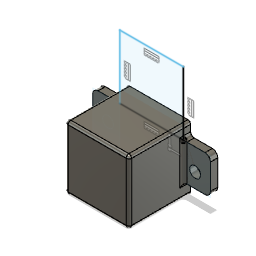
12v ouput cover v1 (Autodesk Fusion 360 design; units mm, degrees)
Autodesk Fusion 360 part; units mm, degrees
sketch "Sketch5" plane through (0, 0, 0) normal (0, 0, 1) x (1, 0, 0)
  line L0 (25.1413, 25.1399) -> (-9.8587, 25.1399)
  line L1 (-9.8587, 25.1399) -> (-9.8587, -9.8601)
  line L2 (-9.8587, -9.8601) -> (25.1413, -9.8601)
  line L3 (25.1413, -9.8601) -> (25.1413, 25.1399)
  line L4 (-9.8587, 18.1399) -> (-24.8587, 18.1399)
  line L5 (-24.8587, 18.1399) -> (-24.8587, -1.8601)
  line L6 (-24.8587, -1.8601) -> (-9.8587, -1.8601)
  line L7 (-9.8587, -1.8601) -> (-9.8587, 18.1399)
  line L8 (25.1413, 18.1399) -> (40.1413, 18.1399)
  line L9 (40.1413, 18.1399) -> (40.1413, -1.8601)
  line L10 (40.1413, -1.8601) -> (25.1413, -1.8601)
  line L11 (25.1413, -1.8601) -> (25.1413, 18.1399)
  dimension "d12" = 35
  dimension "d13" = 35
  dimension "d14" = 15
  dimension "d15" = 20
  dimension "d16" = 7
  dimension "d17" = 15
  dimension "d18" = 20
  dimension "d19" = 7
  constraint horizontal L0
  constraint vertical L1
  constraint horizontal L2
  constraint vertical L3
  constraint horizontal L4
  constraint vertical L5
  constraint horizontal L6
  constraint vertical L7
  constraint coincident L1 L4.start
  constraint horizontal L8
  constraint vertical L9
  constraint horizontal L10
  constraint vertical L11
  constraint coincident L3 L8.start
  measures "d12" distance of L0.start L0.end
  measures "d13" distance of L0.start L2.end
  measures "d14" distance of L4.start L4.end
  measures "d15" distance of L4.start L6.end
  measures "d16" distance of L0 L4
  measures "d17" distance of L8.start L8.end
  measures "d18" distance of L8.start L10.end
  measures "d19" distance of L0 L8
extrude "Extrude4" add sketch "Sketch5" along normal blind 4
sketch "Sketch6" plane through (0, 0, 4) normal (0, 0, 1) x (1, 0, 0)
  line L0 (25.1413, 18.1399) -> (25.1413, 25.1399)
  line L1 (25.1413, 25.1399) -> (-9.8587, 25.1399)
  line L2 (-9.8587, 25.1399) -> (-9.8587, 18.1399)
  line L3 (-9.8587, 18.1399) -> (-24.8587, 18.1399)
  line L4 (-24.8587, 18.1399) -> (-24.8587, -1.8601)
  line L5 (-24.8587, -1.8601) -> (-9.8587, -1.8601)
  line L6 (-9.8587, -1.8601) -> (-9.8587, -9.8601)
  line L7 (-9.8587, -9.8601) -> (25.1413, -9.8601)
  line L8 (25.1413, -9.8601) -> (25.1413, -1.8601)
  line L9 (25.1413, -1.8601) -> (40.1413, -1.8601)
  line L10 (40.1413, -1.8601) -> (40.1413, 18.1399)
  line L11 (40.1413, 18.1399) -> (25.1413, 18.1399)
  circle A0 centre (-16.3587, 6.1399) radius 3
  circle A1 centre (31.6413, 6.1399) radius 3
  line L12 (7.6413, 25.1399) -> (7.6413, -9.8601) construction
  dimension "d22" = 6
  dimension "d23" = 6
  dimension "d24" = 48
  dimension "d25" = 12
  dimension "d26" = 12
  dimension "d27" = 24
  constraint midpoint L1 L12.start
  constraint midpoint L7 L12.end
  measures "d22" diameter of A0
  measures "d23" diameter of A1
  measures "d24" horizontal distance of A0.centre A1.centre
  measures "d25" distance of L3 A0.centre
  measures "d26" distance of L11 A1.centre
  measures "d27" distance of A0.centre L12
extrude "Extrude5" cut sketch "Sketch6" against normal up to surface (4 mm away) contours A0 | A1
sketch "Sketch7" plane through (0, 0, 4) normal (0, 0, 1) x (1, 0, 0)
  circle A0 centre (-16.3587, 6.1399) radius 3
  circle A1 centre (31.6413, 6.1399) radius 3
  line L0 (25.1413, 18.1399) -> (25.1413, 25.1399)
  line L1 (25.1413, 25.1399) -> (-9.8587, 25.1399)
  line L2 (-9.8587, 25.1399) -> (-9.8587, 18.1399)
  line L3 (-9.8587, 18.1399) -> (-24.8587, 18.1399)
  line L4 (-24.8587, 18.1399) -> (-24.8587, -1.8601)
  line L5 (-24.8587, -1.8601) -> (-9.8587, -1.8601)
  line L6 (-9.8587, -1.8601) -> (-9.8587, -9.8601)
  line L7 (-9.8587, -9.8601) -> (25.1413, -9.8601)
  line L8 (25.1413, -9.8601) -> (25.1413, -1.8601)
  line L9 (25.1413, -1.8601) -> (40.1413, -1.8601)
  line L10 (40.1413, -1.8601) -> (40.1413, 18.1399)
  line L11 (40.1413, 18.1399) -> (25.1413, 18.1399)
  line L12 (-5.8587, 21.1399) -> (21.1413, 21.1399)
  line L13 (21.1413, 21.1399) -> (21.1413, -9.8601)
  line L14 (21.1413, -9.8601) -> (-5.8587, -9.8601)
  line L15 (-5.8587, -9.8601) -> (-5.8587, 21.1399)
  dimension "d30" = 4
  dimension "d31" = 4
  dimension "d32" = 4
  constraint coincident L7 L13.end
  measures "d30" distance of L1 L12
  measures "d31" distance of L2 L15
  measures "d32" distance of L0 L13
sketch "Sketch9" plane through (0, 0, 4) normal (0, 0, 1) x (1, 0, 0)
  circle A0 centre (-16.3587, 6.1399) radius 3
  circle A1 centre (31.6413, 6.1399) radius 3
  line L0 (25.1413, 18.1399) -> (25.1413, 25.1399)
  line L1 (25.1413, 25.1399) -> (-9.8587, 25.1399)
  line L2 (-9.8587, 25.1399) -> (-9.8587, 18.1399)
  line L3 (-9.8587, 18.1399) -> (-24.8587, 18.1399)
  line L4 (-24.8587, 18.1399) -> (-24.8587, -1.8601)
  line L5 (-24.8587, -1.8601) -> (-9.8587, -1.8601)
  line L6 (-9.8587, -1.8601) -> (-9.8587, -9.8601)
  line L7 (-9.8587, -9.8601) -> (25.1413, -9.8601)
  line L8 (25.1413, -9.8601) -> (25.1413, -1.8601)
  line L9 (25.1413, -1.8601) -> (40.1413, -1.8601)
  line L10 (40.1413, -1.8601) -> (40.1413, 18.1399)
  line L11 (40.1413, 18.1399) -> (25.1413, 18.1399)
  line L12 (-9.8587, 25.1399) -> (25.1413, 25.1399)
  line L13 (25.1413, 25.1399) -> (25.1413, -9.8601)
  line L14 (25.1413, -9.8601) -> (-9.8587, -9.8601)
  line L15 (-9.8587, -9.8601) -> (-9.8587, 25.1399)
  constraint horizontal L12
  constraint vertical L13
  constraint horizontal L14
  constraint vertical L15
  constraint coincident L7.end L8.start
  constraint coincident L1.end L2.start
extrude "Extrude7" add sketch "Sketch9" along normal blind 30 contours L0 L1 L2 L6 L7 L8 L12 L13 L14 L15
extrude "Extrude6" cut sketch "Sketch7" against normal blind 4 contours L7 L12 L13 L14 L15
sketch "Sketch8" plane through (0, 0, 4) normal (0, 0, 1) x (1, 0, 0)
  line L0 (25.1413, 18.1399) -> (25.1413, -1.8601)
  line L1 (25.1413, -1.8601) -> (40.1413, -1.8601)
  line L2 (40.1413, -1.8601) -> (40.1413, 18.1399)
  line L3 (40.1413, 18.1399) -> (25.1413, 18.1399)
  line L4 (-9.8587, 18.1399) -> (-24.8587, 18.1399)
  line L5 (-24.8587, 18.1399) -> (-24.8587, -1.8601)
  line L6 (-24.8587, -1.8601) -> (-9.8587, -1.8601)
  line L7 (-9.8587, -1.8601) -> (-9.8587, 18.1399)
  circle A0 centre (-16.3587, 6.1399) radius 3
  circle A1 centre (31.6413, 6.1399) radius 3
  line L8 (-9.8587, 53.1399) -> (25.1413, 53.1399)
  line L9 (25.1413, 53.1399) -> (25.1413, 18.1399)
  line L10 (25.1413, 18.1399) -> (-9.8587, 18.1399)
  line L11 (-9.8587, 18.1399) -> (-9.8587, 53.1399)
  constraint horizontal L8
  constraint vertical L9
  constraint horizontal L10
  constraint vertical L11
  constraint coincident L0.start L3.end
sketch "Sketch10" plane through (0, 0, 4) normal (0, 0, -1) x (-1, 0, 0)
  line L0 (-21.1413, -9.8601) -> (5.8587, -9.8601)
  line L1 (5.8587, -9.8601) -> (5.8587, 21.1399)
  line L2 (5.8587, 21.1399) -> (-21.1413, 21.1399)
  line L3 (-21.1413, 21.1399) -> (-21.1413, -9.8601)
  line L4 (-21.1413, 21.1399) -> (5.8587, 21.1399)
  line L5 (5.8587, 21.1399) -> (5.8587, -9.8601)
  line L6 (5.8587, -9.8601) -> (-21.1413, -9.8601)
  line L7 (-21.1413, -9.8601) -> (-21.1413, 21.1399)
  constraint horizontal L4
  constraint vertical L5
  constraint horizontal L6
  constraint vertical L7
  constraint coincident L0.end L1.start
  constraint coincident L2.end L3.start
extrude "Extrude8" cut sketch "Sketch10" against normal up to surface (26 mm away)
fillet "Fillet1" radius 1.5 8 edges at (25.1413, 25.1399, 17) (7.6413, 25.1399, 34) (25.1413, 7.6399, 34) (-9.8587, 7.6399, 34) (-9.8587, 25.1399, 17) (25.1413, -9.8601, 17) (7.6413, -9.8601, 34) (-9.8587, -9.8601, 17)
fillet "Fillet2" radius 2 1 edges at (-9.8587, 8.1399, 4)
fillet "Fillet3" radius 2 1 edges at (-9.8587, 18.1399, 3)
fillet "Fillet4" radius 2 1 edges at (25.1413, 8.1399, 4)
fillet "Fillet5" radius 2 1 edges at (25.1413, 18.1399, 3)
fillet "Fillet6" radius 2 1 edges at (25.1413, -1.8601, 3)
fillet "Fillet7" radius 2 1 edges at (-9.8587, -1.8601, 3)
fillet "Fillet8" radius 3 1 edges at (40.1413, 18.1399, 2)
fillet "Fillet9" radius 3 1 edges at (40.1413, -1.8601, 2)
fillet "Fillet10" radius 3 1 edges at (-24.8587, 18.1399, 2)
fillet "Fillet11" radius 3.5 1 edges at (-24.8587, -1.8601, 2)
